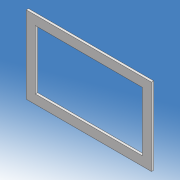
# Autodesk Inventor part: Velcro strip
Saved by Autodesk Inventor 2020 (Build 240168000, 168)
## iProperties
Created: 2019-10-09
Part Number: Velcro strip
Material: Generic
Document SubType Name: Modeling
Designer: mpark
Density: 1 g/cm^3
Appearance: Default
Author: mpark
Autodesk Inventor part; units mm, degrees
ref_plane "YZ Plane" through (0, 0, 0) normal (1, 0, 0) x (0, 1, 0)
ref_plane "XZ Plane" through (0, 0, 0) normal (0, 1, 0) x (-1, 0, 0)
ref_plane "XY Plane" through (0, 0, 0) normal (0, 0, 1) x (1, 0, 0)
sketch "Sketch1" plane through (0, 0, 0) normal (0, 0, 1) x (1, 0, 0)
  line L0 (0, 0) -> (0, 25.4) projected
  line L1 (0, 25.4) -> (-298.45, 25.4) projected
  line L2 (-298.45, 0) -> (-298.45, 25.4) projected
  line L3 (0, 0) -> (-298.45, 0) projected
  line L4 (-323.85, 0) -> (-298.45, 0) projected
  line L5 (-298.45, 0) -> (-298.45, 215.9) projected
  line L6 (-323.85, 215.9) -> (-298.45, 215.9) projected
  line L7 (-323.85, 0) -> (-323.85, 215.9) projected
  line L8 (-298.45, 215.9) -> (-298.45, 190.5) projected
  line L9 (-298.45, 190.5) -> (0, 190.5) projected
  line L10 (0, 215.9) -> (0, 190.5) projected
  line L11 (-298.45, 215.9) -> (0, 215.9) projected
  line L12 (25.4, 215.9) -> (0, 215.9) projected
  line L13 (0, 215.9) -> (0, 0) projected
  line L14 (25.4, 0) -> (0, 0) projected
  line L15 (25.4, 215.9) -> (25.4, 0) projected
  line L16 (-323.85, 0) -> (25.4, 0)
  line L17 (25.4, 0) -> (25.4, 215.9)
  line L18 (25.4, 215.9) -> (-323.85, 215.9)
  line L19 (-323.85, 215.9) -> (-323.85, 0)
  line L20 (0, 25.4) -> (-298.45, 25.4)
  line L21 (-298.45, 25.4) -> (-298.45, 190.5)
  line L22 (-298.45, 190.5) -> (0, 190.5)
  line L23 (0, 190.5) -> (0, 25.4)
  dimension "d0" = 25.4
  dimension "d1" = 25.4
  dimension "d2" = 215.9
  dimension "d3" = 25.4
  dimension "d4" = 25.4
  constraints: 16 end point, 4 parallel, 2 perpendicular, 1 horizontal, 3 other
  measures "d0" distance between parallel lines of L18 L9
  measures "d1" distance between parallel lines of L17 L13
  measures "d2" distance between parallel lines of L18 L16
  measures "d3" distance between parallel lines of L5 L19
  measures "d4" distance between parallel lines of L16 L20
extrude "Extrusion1" add sketch "Sketch1" along normal blind 6.35 contours L3 L2 L1 L0 | L0 L13 L10 L12 L15 L14 | L4 L7 L6 L5 L2 | L9 L5 L11 L10
body "Solid1"
